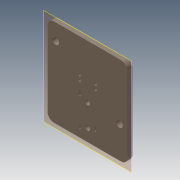
# Autodesk Inventor part: HbSensorBoard01
Saved by Autodesk Inventor 2015 SP1 (Build 190203100, 203)
## iProperties
Created: 2015-05-21
Part Number: HbSensorBoard01
Material: Generic
Document SubType Name: Modeling
Designer: Yamaura
Density: 1 g/cm^3
Appearance: Default
Author: Yamaura
Autodesk Inventor part; units mm, degrees
ref_plane "YZ Plane" through (0, 0, 0) normal (1, 0, 0) x (0, 1, 0)
ref_plane "XZ Plane" through (0, 0, 0) normal (0, 1, 0) x (-1, 0, 0)
ref_plane "XY Plane" through (0, 0, 0) normal (0, 0, 1) x (1, 0, 0)
ref_plane "作業平面1" through (0, 0, 0) normal (0, 0, 1) x (1, 0, 0)
sketch "スケッチ1" plane through (0, 0, 0) normal (0, 0, 1) x (1, 0, 0)
  line L0 (-12.7, 11.83) -> (-12.7, 13.57) projected
  line L1 (-12.3, 13.97) -> (-10.56, 13.97) projected
  line L2 (12.3, -13.97) -> (10.56, -13.97) projected
  line L3 (12.7, -11.83) -> (12.7, -13.57) projected
  line L4 (-12.7, 13.97) -> (12.7, 13.97)
  line L5 (12.7, 13.97) -> (12.7, -13.97)
  line L6 (12.7, -13.97) -> (-12.7, -13.97)
  line L7 (-12.7, -13.97) -> (-12.7, 13.97)
  point P0 (0, 0)
  constraints: 8 end point, 2 parallel, 1 horizontal, 1 perpendicular, 1 point on line
extrude "押し出し1" add sketch "スケッチ1" against normal blind 1.6
sketch "スケッチ2" plane through (0, 0, 0) normal (0, 0, 1) x (1, 0, 0)
  circle A0 centre (-10.16, 8.89) radius 1.1
  circle A1 centre (10.16, -3.81) radius 1.1
  point P0 (0, 0)
  dimension "d2" = 2.2
  dimension "d3" = 2.2
  dimension "d4" = 10.16
  dimension "d5" = 8.89
  dimension "d6" = 3.81
  dimension "d7" = 10.16
  constraints: 2 centre point
  measures "d2" diameter of A0
  measures "d3" diameter of A1
  measures "d4" horizontal distance of point (0, 0) A0.centre
  measures "d5" vertical distance of point (0, 0) A0.centre
  measures "d6" vertical distance of A1.centre point (0, 0)
  measures "d7" horizontal distance of A1.centre point (0, 0)
extrude "押し出し2" cut sketch "スケッチ2" along normal mid plane 20
sketch "スケッチ3" plane through (0, 0, 0) normal (0, 0, 1) x (1, 0, 0)
  circle A0 centre (-2.54, 3.81) radius 0.4 projected
  circle A1 centre (-2.54, 1.27) radius 0.4 projected
  circle A2 centre (2.54, 3.81) radius 0.4 projected
  circle A3 centre (2.54, 1.27) radius 0.4 projected
  point P0 (0, 0)
extrude "押し出し3" cut sketch "スケッチ3" along normal mid plane 20
sketch "スケッチ4" plane through (0, 0, 0) normal (0, 0, 1) x (1, 0, 0)
  circle A0 centre (-2.54, 1.27) radius 0.4 projected
  circle A1 centre (-2.54, 3.81) radius 0.4 projected
  circle A2 centre (2.54, 1.27) radius 0.4 projected
  circle A3 centre (2.54, 3.81) radius 0.4 projected
  circle A4 centre (0, 2.54) radius 0.05
  line L0 (0, -30.1689) -> (0, 24.3248)
  point P0 (0, 0)
  dimension "d12" = 0.1
  dimension "d13" = 2.54
  constraints: 2 end point, 1 centre point, 1 coincident, 1 point on line, 1 vertical, 2 other
  measures "d12" diameter of A4
  measures "d13" distance of point (0, 2.54) point (0, 0)
extrude "押し出し4" cut sketch "スケッチ4" against normal blind 20 contours A4 L0 | L0 A4
sketch "スケッチ5" plane through (0, 0, 0) normal (0, 0, 1) x (1, 0, 0)
  circle A0 centre (0, -3) radius 0.8
  circle A1 centre (0, -10) radius 0.8
  point P0 (0, 0)
  dimension "d16" = 1.6
  dimension "d17" = 1.6
  dimension "d18" = 3
  dimension "d19" = 7
  constraints: 2 centre point
  measures "d16" diameter of A0
  measures "d17" diameter of A1
  measures "d18" distance of A0.centre point (0, 0)
  measures "d19" distance of A1.centre A0.centre
extrude "押し出し5" cut sketch "スケッチ5" against normal blind 20
sketch "スケッチ6" plane through (0, 0, 0) normal (0, 0, 1) x (1, 0, 0)
  line L0 (-2.55, -1.3) -> (-2.35, -1.3) projected
  line L1 (-2.55, -1.3) -> (-2.55, -1.8) projected
  line L2 (-2.35, -1.8) -> (-2.55, -1.8) projected
  line L3 (-2.35, -1.8) -> (-2.35, -1.3) projected
  line L4 (2.55, -8.6) -> (2.55, -9.6) projected
  line L5 (2.35, -9.6) -> (2.35, -8.6) projected
  line L6 (-2.35, -10.4) -> (-2.35, -11.4) projected
  circle A0 centre (0, -3) radius 0.8 projected
  circle A1 centre (0, -10) radius 0.8 projected
  circle A2 centre (0, 2.54) radius 0.05 projected
  circle A3 centre (2.54, 3.81) radius 0.4 projected
  circle A4 centre (-2.54, 3.81) radius 0.4 projected
  circle A5 centre (-2.54, 1.27) radius 0.4 projected
  circle A6 centre (2.54, 1.27) radius 0.4 projected
  circle A7 centre (-10.16, 8.89) radius 1.1 projected
  circle A8 centre (10.16, -3.81) radius 1.1 projected
  line L7 (-12.7, 13.97) -> (12.7, 13.97) projected
  line L8 (-12.7, -13.97) -> (-12.7, 13.97) projected
  line L9 (12.7, -13.97) -> (-12.7, -13.97) projected
  line L10 (12.7, 13.97) -> (12.7, -13.97) projected
  line L11 (-2.55, -11.4) -> (-2.55, -10.4) projected
  line L12 (-2.35, -1.8) -> (-2.35, -2.3) projected
  line L13 (-2.55, -2.3) -> (-2.55, -1.8) projected
  line L14 (-2.35, -0.8) -> (-2.35, -1.3) projected
  line L15 (-2.55, -1.3) -> (-2.55, -0.8) projected
  line L16 (-2.55, -1.3) -> (-2.35, -1.8)
  line L17 (2.35, -8.6) -> (2.55, -9.6)
  line L18 (-2.55, -10.4) -> (-2.35, -11.4)
  line L19 (-2.55, -0.8) -> (-2.35, -0.8)
  line L20 (-2.55, -2.3) -> (-2.35, -2.3)
  line L21 (2.35, -8.6) -> (2.55, -8.6)
  line L22 (2.55, -9.6) -> (2.35, -9.6)
  line L23 (-2.55, -10.4) -> (-2.35, -10.4)
  line L24 (-2.55, -11.4) -> (-2.35, -11.4)
  line L25 (-2.45, -2.3) -> (-2.45, -0.8) construction
  line L26 (-2.2, -2.3) -> (-2.2, -0.8)
  line L27 (-2.7, -0.8) -> (-2.7, -2.3)
  arc A9 (-2.7, -2.3) -> (-2.2, -2.3) centre (-2.45, -2.3) ccw
  arc A10 (-2.2, -0.8) -> (-2.7, -0.8) centre (-2.45, -0.8) ccw
  line L28 (2.45, -9.6) -> (2.45, -8.6) construction
  line L29 (2.7, -9.6) -> (2.7, -8.6)
  line L30 (2.2, -8.6) -> (2.2, -9.6)
  arc A11 (2.2, -9.6) -> (2.7, -9.6) centre (2.45, -9.6) ccw
  arc A12 (2.7, -8.6) -> (2.2, -8.6) centre (2.45, -8.6) ccw
  line L31 (-2.45, -11.4) -> (-2.45, -10.4) construction
  line L32 (-2.2, -11.4) -> (-2.2, -10.4)
  line L33 (-2.7, -10.4) -> (-2.7, -11.4)
  arc A13 (-2.7, -11.4) -> (-2.2, -11.4) centre (-2.45, -11.4) ccw
  arc A14 (-2.2, -10.4) -> (-2.7, -10.4) centre (-2.45, -10.4) ccw
  point P0 (0, 0)
  point P1 (-2.45, -1.55)
  point P2 (2.45, -9.1)
  point P3 (-2.45, -10.9)
  dimension "d22" = 0.2
  dimension "d23" = 0.5
  dimension "d24" = 0.5
  dimension "d25" = 0.5
  constraints: 42 end point, 12 point on circle, 12 tangent, 9 midpoint, 8 parallel, 6 centre point, 2 horizontal
  measures "d22" distance of L2.start L1.end
  measures "d23" diameter of A10
  measures "d24" diameter of A12
  measures "d25" diameter of A14
extrude "押し出し6" cut sketch "スケッチ6" against normal blind 2 contours L15 L19 L14 L0 | L16 L2 L1 | L0 L3 L16 | L2 L12 L20 L13 | L4 L17 L21 | L22 L5 L17 | L6 L18 L23 | L24 L11 L18 | A9 L27 A10 L26 | A11 L30 A12 L29 | A13 L33 A14 L32
fillet "フィレット1" radius 2 4 edges at (-12.7, -13.97, -0.8) (12.7, -13.97, -0.8) (12.7, 13.97, -0.8) (-12.7, 13.97, -0.8)
move faces "移動1" translate (0, 0.52, 0) faces at (-2.1452, 1.2058, -0.5333) (2.9348, 1.2058, -0.5333)
move faces "移動2" translate (0, -0.52, 0) faces at (-2.1452, 3.7458, -0.5333) (2.9348, 3.7458, -0.5333)
